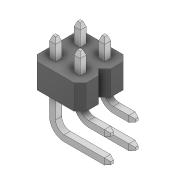
# Autodesk Inventor part: 2pin_header
Saved by Autodesk Inventor 2020 (Build 240168000, 168)
## iProperties
Created: 2023-02-11
Part Number: 2pin_header
Material: 일반
Document SubType Name: Modeling
Designer: OFFLINE
Density: 1 g/cm^3
Appearance: 기본값
Author: OFFLINE
Autodesk Inventor part; units mm, degrees
ref_plane "YZ Plane" through (0, 0, 0) normal (1, 0, 0) x (0, 1, 0)
ref_plane "XZ Plane" through (0, 0, 0) normal (0, 1, 0) x (-1, 0, 0)
sketch "스케치1" plane through (0, 0, 0) normal (0, 0, 1) x (1, 0, 0)
  line L0 (4.6, 1.75) -> (2.95, 1.75)
  line L1 (1.75, 2.95) -> (1.75, 6.65)
  line L2 (-0.25, 6.65) -> (-0.25, 0.95)
  line L3 (0.95, -0.25) -> (4.6, -0.25)
  arc A0 (-0.25, 0.95) -> (0.95, -0.25) centre (0.95, 0.95) ccw
  line L4 (0.25, 6.65) -> (0.25, 0.95)
  arc A1 (0.25, 0.95) -> (0.95, 0.25) centre (0.95, 0.95) ccw
  line L5 (0.95, 0.25) -> (4.6, 0.25)
  arc A2 (1.75, 2.95) -> (2.95, 1.75) centre (2.95, 2.95) ccw
  line L6 (2.25, 6.65) -> (2.25, 2.95)
  arc A3 (2.25, 2.95) -> (2.95, 2.25) centre (2.95, 2.95) ccw
  line L7 (2.95, 2.25) -> (4.6, 2.25)
  line L8 (-0.25, 6.65) -> (0.25, 6.65)
  line L9 (1.75, 6.65) -> (2.25, 6.65)
  line L10 (4.6, 2.25) -> (4.6, 1.75)
  line L11 (4.6, 0.25) -> (4.6, -0.25)
  point P0 (0, 0)
  point P1 (1.75, 1.75)
  point P2 (-0.25, -0.25)
  dimension "d12" = 1.2
  dimension "d13" = 0.5
  dimension "d14" = 1.2
  dimension "d15" = 0.5
  constraints: 24 end point, 8 point on circle, 4 centre point, 4 point on line, 4 tangent, 2 collinear, 1 horizontal, 1 perpendicular
  measures "d12" radius of A0
  measures "d13" distance between parallel lines of L2 L4
  measures "d14" radius of A2
  measures "d15" distance between parallel lines of L1 L6
extrude "돌출1" add sketch "스케치1" along normal blind 0.5
ref_plane "작업 평면1" through (0.95, 3.05, 0) normal (0, -1, 0) x (1, 0, 0)
sketch "스케치2" plane through (0.95, 3.05, 0) normal (0, -1, 0) x (1, 0, 0)
  line L0 (-1.2, 0) -> (0, 0) projected
  line L1 (0, 0) -> (0, 0.5) projected
  line L2 (-1.2, 0.5) -> (0, 0.5) projected
  line L3 (-1.2, 0) -> (-1.2, 0.5) projected
  line L4 (0, 0.5) -> (3.65, 0.5) projected
  line L5 (0, 0) -> (0, 0.5) projected
  line L6 (0, 0) -> (3.65, 0) projected
  line L7 (0.94, 0.14) -> (1.16, 0.14) projected
  line L8 (0.94, 0.36) -> (0.94, 0.14) projected
  line L9 (1.16, 0.36) -> (0.94, 0.36) projected
  line L10 (1.16, 0.14) -> (1.16, 0.36) projected
  line L11 (-0.7, 0) -> (-1.2, 0) projected
  line L12 (-1.2, 0) -> (1.3, 0)
  line L13 (1.3, 0) -> (1.3, 0.5)
  line L14 (1.3, 0.5) -> (-1.2, 0.5)
  line L15 (-1.2, 0.5) -> (-1.2, 0)
  line L16 (-1.95, 1.25) -> (2.05, 1.25)
  line L17 (2.05, 1.25) -> (2.05, -0.75)
  line L18 (2.05, -0.75) -> (-1.95, -0.75)
  line L19 (-1.95, -0.75) -> (-1.95, 1.25)
  line L20 (-0.7, 0) -> (-0.7, 0.5) projected
  line L21 (-1.2, 0) -> (-1.2, 0.5) projected
  line L22 (-0.7, 0) -> (-1.2, 0) projected
  line L23 (-0.7, 0.5) -> (-1.2, 0.5) projected
  line L24 (3.65, 0) -> (3.65, 0.5) projected
  point P0 (-0.95, 0)
  dimension "d36" = 0.75
  constraints: 16 end point, 4 parallel, 2 perpendicular, 1 horizontal, 3 other
  measures "d36" distance between parallel lines of L14 L16
extrude "돌출2" add sketch "스케치2" against normal blind 2 contours L3 L2 L20 L0 | L0 L6 L17 L18 L19 L16 L4 L2 L3 | L20 L2 L1 L0 | L1 L4 L13 L6 | L13 L4 L17 L6 | L8 L9 L10 L7
chamfer "모따기7" distance 0.14 angle 70 4 edges at (0, 6.65, 0.5) (-0.25, 6.65, 0.25) (0, 6.65, 0) (0.25, 6.65, 0.25) measured on face at (0.0833, 6.65, 0.1667)
chamfer "모따기8" distance 0.14 angle 70 4 edges at (1.75, 6.65, 0.25) (2, 6.65, 0) (2.25, 6.65, 0.25) (2, 6.65, 0.5) measured on face at (2.0833, 6.65, 0.1667)
chamfer "모따기9" distance 0.14 angle 70 4 edges at (4.6, 2, 0.5) (4.6, 2.25, 0.25) (4.6, 2, 0) (4.6, 1.75, 0.25) measured on face at (4.6, 1.9167, 0.1667)
chamfer "모따기10" distance 0.14 angle 70 4 edges at (4.6, 0.25, 0.25) (4.6, 0, 0.5) (4.6, 0, 0) (4.6, -0.25, 0.25) measured on face at (4.6, -0.0833, 0.1667)
chamfer "모따기11" distance 0.5 angle 45 4 edges at (-1, 4.05, 1.25) (3, 4.05, 1.25) (3, 4.05, -0.75) (-1, 4.05, -0.75)
pattern_linear "직사각형 패턴1" count 2 spacing 2 along (0, 0, 1) of "돌출1", "돌출2", "모따기7", "모따기8", "모따기9", "모따기10", "모따기11"
ref_plane "작업 평면2" through (0.95, 3.05, 2) normal (0, -1, 0) x (1, 0, 0)
